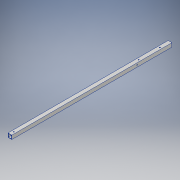
# Autodesk Inventor part: bepf_glowny_wspornik
Saved by Autodesk Inventor 2017 (Build 210142000, 142)
## iProperties
Created: 2016-11-24
Part Number: bepf_glowny_wspornik
Material: Aluminium 6061
Document SubType Name: Modeling
Designer: gagato
Density: 2.7 g/cm^3
Appearance: Aluminium — płaski
Mass: 137.547 g
Surface Area: 681.855 cm^2
Volume: 50.9434 cm^3
Author: gagato
Autodesk Inventor part; units mm, degrees
ref_plane "YZ Plane" through (0, 0, 0) normal (1, 0, 0) x (0, 1, 0)
ref_plane "XZ Plane" through (0, 0, 0) normal (0, 1, 0) x (-1, 0, 0)
ref_plane "XY Plane" through (0, 0, 0) normal (0, 0, 1) x (1, 0, 0)
sketch "Szkic1" plane through (0, 0, 0) normal (0, 1, 0) x (-1, 0, 0)
  line L0 (-7.5, -7.5) -> (7.5, -7.5)
  line L1 (7.5, -7.5) -> (7.5, 7.5)
  line L2 (7.5, 7.5) -> (-7.5, 7.5)
  line L3 (-7.5, 7.5) -> (-7.5, -7.5)
  line L4 (-7.5, -7.5) -> (7.5, 7.5) construction
  line L5 (7.5, -7.5) -> (-7.5, 7.5) construction
  line L6 (6, -6) -> (-6, -6)
  line L7 (-6, -6) -> (-6, 6)
  line L8 (-6, 6) -> (6, 6)
  line L9 (6, 6) -> (6, -6)
  line L10 (6, -6) -> (-6, 6) construction
  line L11 (-6, -6) -> (6, 6) construction
  point P0 (0, 0)
  dimension "d0" = 15
  dimension "d1" = 15
  dimension "d2" = 12
  dimension "d3" = 12
  constraints: 24 end point, 4 midpoint, 4 parallel, 2 horizontal, 2 perpendicular
  measures "d0" distance of L2.end L1.end
  measures "d1" distance of L1.end L0.end
  measures "d2" distance of L7.end L8.end
  measures "d3" distance of L6.end L7.end
extrude "Wyciągnięcie proste1" add sketch "Szkic1" along normal blind 630
sketch "Szkic2" plane through (-7.5, 0, 7.5) normal (0, 0, 1) x (1, 0, 0)
  line L0 (7.5, 0) -> (7.5, 15) construction
  dimension "d6" = 15
  constraints: 2 end point, 1 coincident, 1 vertical
  measures "d6" distance of L0.start L0.end
hole "Otwór1" at (0, 15, 7.5) direction (0, 0, -1) diameter 3.5 end through all
sketch "Szkic3" plane through (7.5, 0, 7.5) normal (1, 0, 0) x (0, 0, -1)
  line L0 (13.5, 630) -> (1.5, 630) construction
  line L1 (7.5, 630) -> (7.5, 492.75) construction
  point P0 (7.5, 0)
  dimension "d14" = 137.25
  constraints: 2 end point, 1 coincident, 1 midpoint, 1 vertical
  measures "d14" distance of L1.start L1.end
hole "Otwór2" at (7.5, 492.75, 0) direction (-1, 0, 0) diameter 3.5 end through all
sketch "Szkic4" plane through (-7.5, 0, 7.5) normal (0, 0, 1) x (1, 0, 0)
  line L0 (13.5, 630) -> (1.5, 630) construction
  line L1 (7.5, 630) -> (7.5, 590) construction
  line L2 (7.5, 630) -> (7.5, 506.5) construction
  point P0 (7.5, 0)
  dimension "d22" = 40
  dimension "d32" = 123.5
  constraints: 4 end point, 2 coincident, 1 midpoint, 1 point on line, 1 vertical
  measures "d22" distance of L1.start L1.end
  measures "d32" distance of L1.start L2.end
hole "Otwór3" at (0, 590, 7.5) at (0, 506.5, 7.5) direction (0, 0, -1) diameter 3.5 end through all
